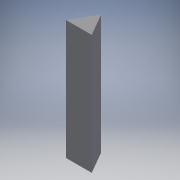
# Autodesk Inventor part: alignmentPin
Saved by Autodesk Inventor 2017 (Build 210142000, 142)
## iProperties
Created: 2016-11-02
Part Number: alignmentPin
Material: Generic
Document SubType Name: Modeling
Designer: Camilo
Density: 1 g/cm^3
Appearance: Default
Author: Camilo
Autodesk Inventor part; units mm, degrees
ref_plane "YZ Plane" through (0, 0, 0) normal (1, 0, 0) x (0, 1, 0)
ref_plane "XZ Plane" through (0, 0, 0) normal (0, 1, 0) x (-1, 0, 0)
ref_plane "XY Plane" through (0, 0, 0) normal (0, 0, 1) x (1, 0, 0)
sketch "Sketch1" plane through (0, 0, 0) normal (0, 0, 1) x (1, 0, 0)
  line L0 (5.0151, 1.7783) -> (2.5151, 1.7783) construction
  line L1 (3.7651, 3.9434) -> (5.0151, 1.7783) construction
  line L2 (2.5151, 1.7783) -> (3.7651, 3.9434) construction
  line L3 (2.6883, 1.8783) -> (4.8419, 1.8783)
  line L4 (4.8419, 1.8783) -> (3.7651, 3.7434)
  line L5 (3.7651, 3.7434) -> (2.6883, 1.8783)
  point P0 (0, 0)
  dimension "d0" = 0.1
  constraints: 6 end point, 2 other
  measures "d0" distance between parallel lines of L0 L3
extrude "Extrusion1" add sketch "Sketch1" along normal mid plane 10
body "Solid1"
